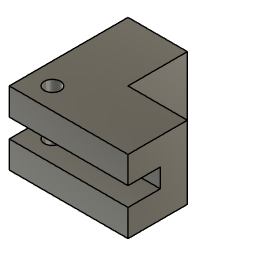
hammockHolder v1 (Autodesk Fusion 360 design; units mm, degrees)
Autodesk Fusion 360 part; units mm, degrees
sketch "Sketch1" plane through (0, 0, 0) normal (0, 0, 1) x (1, 0, 0)
  line L0 (0, 0) -> (11, 0)
  line L1 (11, 0) -> (11, 22)
  line L2 (11, 22) -> (0, 22)
  line L3 (0, 22) -> (0, 0)
  line L4 (11, 0) -> (22, 0)
  line L5 (22, 0) -> (22, 11)
  line L6 (22, 11) -> (11, 11)
  line L7 (11, 11) -> (11, 0)
  dimension "d1" = 11
  dimension "d2" = 22
  dimension "d3" = 11
  dimension "d4" = 11
  constraint horizontal L0
  constraint vertical L1
  constraint horizontal L2
  constraint vertical L3
  constraint coincident L0.start L3.end
  constraint horizontal L4
  constraint vertical L5
  constraint horizontal L6
  constraint vertical L7
  measures "d1" distance of L0.start L0.end
  measures "d2" distance of L0.start L2.end
  measures "d3" distance of L0.end L4.end
  measures "d4" distance of L0.end L6.end
extrude "Extrude1" add sketch "Sketch1" along normal blind 5
sketch "Sketch2" plane through (0, 0, 5) normal (0, 0, 1) x (-1, 0, 0)
  line L0 (-22, -11) -> (-11, -11)
  line L1 (-11, -11) -> (-11, -22)
  line L2 (-11, -22) -> (0, -22)
  line L3 (0, -22) -> (0, 0)
  line L4 (0, 0) -> (-22, 0)
  line L5 (-22, 0) -> (-22, -11)
  line L6 (-22, -11) -> (-5.9353, -11)
  line L7 (-5.9353, -11) -> (-5.9353, -5.9846)
  line L8 (-5.9353, -5.9846) -> (-22, -5.9846)
  line L9 (-22, -5.9846) -> (-22, -11)
  line L10 (-5.9353, -22) -> (-11, -22)
  line L11 (-11, -22) -> (-11, -11)
  line L12 (-11, -11) -> (-5.9353, -11)
  line L13 (-5.9353, -11) -> (-5.9353, -22)
  constraint horizontal L6
  constraint vertical L7
  constraint horizontal L8
  constraint vertical L9
  constraint coincident L0.start L5.end
  constraint horizontal L10
  constraint vertical L11
  constraint horizontal L12
  constraint vertical L13
  constraint coincident L0.end L1.start
  constraint coincident L2 L10.start
extrude "Extrude2" add sketch "Sketch2" along normal blind 3.5 contours L0 L5 L6 L7 L8 L9 L12 | L1 L2 L6 L10 L11 L12 L13
sketch "Sketch3" plane through (0, 0, 8.5) normal (0, 0, 1) x (-1, 0, 0)
  line L0 (-5.9353, -5.9846) -> (-22, -5.9846)
  line L1 (-22, -5.9846) -> (-22, -11)
  line L2 (-22, -11) -> (-11, -11)
  line L3 (-11, -11) -> (-11, -22)
  line L4 (-11, -22) -> (-5.9353, -22)
  line L5 (-5.9353, -22) -> (-5.9353, -5.9846)
  line L6 (0, -22) -> (-11, -22)
  line L7 (-11, -22) -> (-11, 0)
  line L8 (-11, 0) -> (0, 0)
  line L9 (0, 0) -> (0, -22)
  line L10 (-11, -11) -> (-22, -11)
  line L11 (-22, -11) -> (-22, 0)
  line L12 (-22, 0) -> (-11, 0)
  line L13 (-11, 0) -> (-11, -11)
  constraint horizontal L6
  constraint vertical L7
  constraint horizontal L8
  constraint vertical L9
  constraint horizontal L10
  constraint vertical L11
  constraint horizontal L12
  constraint vertical L13
  constraint coincident L2.end L3.start
extrude "Extrude3" add sketch "Sketch3" along normal blind 5
sketch "Sketch4" plane through (0, 0, 13.5) normal (0, 0, 1) x (-1, 0, 0)
  line L0 (-22, 0) -> (-22, -11)
  line L1 (-22, -11) -> (-11, -11)
  line L2 (-11, -11) -> (-11, -22)
  line L3 (-11, -22) -> (0, -22)
  line L4 (0, -22) -> (0, 0)
  line L5 (0, 0) -> (-22, 0)
  circle A0 centre (-4, -4) radius 1.5
  dimension "d11" = 3
  measures "d11" diameter of A0
extrude "Extrude4" cut sketch "Sketch4" against normal blind 17 contours A0
